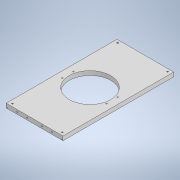
# Autodesk Inventor part: Grundplatte1.0
Saved by Autodesk Inventor 2021.3 (Build 253353000, 353)
## iProperties
Created: 2021-10-11
Part Number: Grundplatte1.0
Material: Generisch
Document SubType Name: Modeling
Designer: bhelg
Density: 1 g/cm^3
Appearance: Vorgabe
Author: bhelg
Autodesk Inventor part; units mm, degrees
ref_plane "YZ Plane" through (0, 0, 0) normal (1, 0, 0) x (0, 1, 0)
ref_plane "XZ Plane" through (0, 0, 0) normal (0, 1, 0) x (-1, 0, 0)
ref_plane "XY Plane" through (0, 0, 0) normal (0, 0, 1) x (1, 0, 0)
sketch "Skizze2" plane through (0, 0, 0) normal (0, 1, 0) x (-1, 0, 0)
  circle A0 centre (0, 0) radius 75
  line L0 (-102.5, -200) -> (102.5, -200)
  line L1 (102.5, -200) -> (102.5, 200)
  line L2 (102.5, 200) -> (-102.5, 200)
  line L3 (-102.5, 200) -> (-102.5, -200)
  line L4 (-102.5, -200) -> (102.5, 200) construction
  line L5 (102.5, -200) -> (-102.5, 200) construction
  dimension "d8" = 150
  dimension "d9" = 205
  dimension "d10" = 400
  constraints: 12 end point, 2 midpoint, 2 parallel, 1 centre point, 1 coincident, 1 horizontal, 1 perpendicular
  measures "d8" diameter of A0
  measures "d9" distance of L2.end L1.end
  measures "d10" distance of L1.end L0.end
extrude "Extrusion1" add sketch "Skizze2" along normal blind 15
sketch "Skizze3" plane through (0, 0, 0) normal (0, -1, 0) x (1, 0, 0)
  line L0 (-90, -190) -> (90, -190)
  line L1 (90, -190) -> (90, 190)
  line L2 (90, 190) -> (-90, 190)
  line L3 (-90, 190) -> (-90, -190)
  line L4 (-90, -190) -> (90, 190) construction
  line L5 (90, -190) -> (-90, 190) construction
  point P0 (0, 0)
  dimension "d13" = 180
  dimension "d14" = 380
  constraints: 12 end point, 2 midpoint, 2 parallel, 1 horizontal, 1 perpendicular
  measures "d13" distance of L2.end L1.end
  measures "d14" distance of L1.end L0.end
hole "Bohrung1" at (90, 0, -190) at (-90, 0, -190) at (-90, 0, 190) at (90, 0, 190) direction (0, 1, 0) diameter 4.917 end through all thread size "M6x1" class "6H" standard "ISO Metric profile"
sketch "Skizze4" plane through (-102.5, 0, 200) normal (0, 0, 1) x (1, 0, 0)
  line L0 (0, 0) -> (0, 15) projected
  line L1 (0, 0) -> (205, 0) projected
  line L2 (205, 0) -> (205, 15) projected
  point P0 (102.5, 0)
  point P1 (40, 7.5)
  point P2 (165, 7.5)
  point P3 (76, 7.5)
  point P4 (129, 7.5)
  dimension "d23" = 40
  dimension "d24" = 7.5
  dimension "d25" = 7.5
  dimension "d44" = 36
  dimension "d45" = 36
  dimension "d46" = 7.5
  dimension "d47" = 7.5
  dimension "d48" = 40
  measures "d23" distance from line of L0 point (40, 7.5)
  measures "d24" distance from line of point (40, 7.5) L1
  measures "d25" distance from line of L1 point (165, 7.5)
  measures "d44" distance of point (76, 7.5) point (40, 7.5)
  measures "d45" distance of point (165, 7.5) point (129, 7.5)
  measures "d46" distance from line of point (76, 7.5) L1
  measures "d47" distance from line of point (129, 7.5) L1
  measures "d48" distance from line of L2 point (165, 7.5)
sketch "Skizze5" plane through (102.5, 0, -200) normal (0, 0, -1) x (-1, 0, 0)
  line L0 (205, 0) -> (205, 15) projected
  line L1 (0, 0) -> (205, 0) projected
  line L2 (0, 0) -> (0, 15) projected
  point P0 (102.5, 0)
  point P1 (40, 7.5)
  point P2 (165, 7.5)
  point P3 (76, 7.5)
  point P4 (129, 7.5)
  dimension "d27" = 40
  dimension "d28" = 7.5
  dimension "d29" = 7.5
  dimension "d49" = 7.5
  dimension "d50" = 7.5
  dimension "d51" = 36
  dimension "d52" = 36
  dimension "d53" = 40
  measures "d27" distance from line of L0 point (165, 7.5)
  measures "d28" distance from line of L1 point (40, 7.5)
  measures "d29" distance from line of L1 point (165, 7.5)
  measures "d49" distance from line of point (76, 7.5) L1
  measures "d50" distance from line of L1 point (129, 7.5)
  measures "d51" distance of point (76, 7.5) point (40, 7.5)
  measures "d52" distance of point (165, 7.5) point (129, 7.5)
  measures "d53" distance from line of point (40, 7.5) L2
hole "Bohrung4" at (62.5, 7.5, -200) at (26.5, 7.5, -200) at (-26.5, 7.5, -200) at (-62.5, 7.5, -200) direction (0, 0, 1) diameter 4.134 depth 14.2 tip angle 118 thread size "M5x0.8" class "6H" standard "ISO Metric profile"
hole "Bohrung5" at (-62.5, 7.5, 200) at (62.5, 7.5, 200) at (-26.5, 7.5, 200) at (26.5, 7.5, 200) direction (0, 0, -1) diameter 4.134 depth 14.2 tip angle 118 thread size "M5x0.8" class "6H" standard "ISO Metric profile"
sketch "Skizze6" plane through (0, 0, 0) normal (0, -1, 0) x (1, 0, 0)
  line L0 (99, 200) -> (99, -200)
  line L1 (102.5, 200) -> (102.5, -200) projected
  line L2 (96.5, 200) -> (96.5, -200)
  line L3 (-99, -200) -> (-99, 200)
  line L4 (-96.5, -200) -> (-96.5, 200)
  line L5 (102.5, -200) -> (-102.5, -200) projected
  line L6 (96.5, -200) -> (99, -200)
  line L7 (-96.5, -200) -> (-99, -200)
  line L8 (-102.5, 200) -> (102.5, 200) projected
  line L9 (-96.5, 200) -> (-99, 200)
  line L10 (99, 200) -> (96.5, 200)
  line L11 (-102.5, -200) -> (-102.5, 200) projected
  point P0 (0, 0)
  point P1 (96.5, 200)
  dimension "d68" = 2.5
  dimension "d70" = 2.5
  dimension "d84" = 198
  dimension "d85" = 99
  constraints: 16 end point, 8 point on line, 2 parallel, 2 vertical
  measures "d68" distance between parallel lines of L2 L0
  measures "d70" distance between parallel lines of L3 L4
  measures "d84" distance between parallel lines of L3 L0
  measures "d85" distance from line of point (0, 0) L0
extrude "Extrusion2" cut sketch "Skizze6" against normal blind 2.5 contours L0 L5 L2 L8 | L4 L5 L3 L8
sketch "Skizze7" plane through (0, 0, 0) normal (0, -1, 0) x (1, 0, 0)
  line L0 (-80, -20) -> (80, -20)
  line L1 (80, -20) -> (80, 20)
  line L2 (80, 20) -> (-80, 20)
  line L3 (-80, 20) -> (-80, -20)
  line L4 (-80, -20) -> (80, 20) construction
  line L5 (80, -20) -> (-80, 20) construction
  point P0 (0, 0)
  dimension "d74" = 160
  dimension "d75" = 40
  constraints: 12 end point, 2 midpoint, 2 parallel, 1 horizontal, 1 perpendicular
  measures "d74" distance of L2.end L1.end
  measures "d75" distance of L0.end L1.end
hole "Bohrung6" at (-80, 0, 20) at (-80, 0, -20) at (80, 0, -20) at (80, 0, 20) direction (0, 1, 0) diameter 4.134 end through all thread size "M5x0.8" class "6H" standard "ISO Metric profile"
equation "\"d70\" = d68"
equation "\"d85\" = 0.5 * d84"
